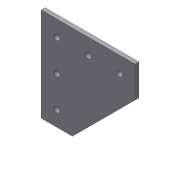
# Autodesk Inventor part: Frame_VerticalAngle_Plate
Saved by Autodesk Inventor 2012 (Build 160160000, 160)
## iProperties
Created: 2012-01-14
Part Number: Frame_VerticalAngle_Plate
Material: Aluminum-6061
Document SubType Name: Modeling
Designer: JesseK
Mass: 38.0914 g
Surface Area: 99.6488 cm^2
Volume: 14.0559 cm^3
Density: 2.71 g/cm^3
Author: JesseK
Autodesk Inventor part; units mm, degrees
ref_plane "YZ Plane" through (0, 0, 0) normal (1, 0, 0) x (0, 1, 0)
ref_plane "XZ Plane" through (0, 0, 0) normal (0, 1, 0) x (-1, 0, 0)
ref_plane "XY Plane" through (0, 0, 0) normal (0, 0, 1) x (1, 0, 0)
sketch "Sketch1" plane through (0, 0, 0) normal (0, 0, 1) x (1, 0, 0)
  line L0 (0, 0) -> (25.4, 0)
  line L1 (25.4, 0) -> (76.2, 50.8)
  line L2 (76.2, 50.8) -> (76.2, 76.2)
  line L3 (76.2, 76.2) -> (0, 76.2)
  line L4 (0, 76.2) -> (0, 0)
  dimension "d0" = 76.2
  dimension "d1" = 76.2
  dimension "d2" = 25.4
  dimension "d3" = 25.4
  constraints: 10 end point, 2 horizontal, 2 vertical
  measures "d0" distance of L2.end L3.end
  measures "d1" distance of L3.end L0.start
  measures "d2" distance of L0.start L0.end
  measures "d3" distance of L1.end L2.end
extrude "Extrusion1" add sketch "Sketch1" along normal blind 3.175
sketch "Sketch2" plane through (0, 0, 3.175) normal (0, 0, 1) x (1, 0, 0)
  line L0 (0, 0) -> (0, 76.2) projected
  line L1 (0, 76.2) -> (76.2, 76.2) projected
  circle A0 centre (12.7, 63.5) radius 2.3813
  dimension "d6" = 4.7625
  dimension "d7" = 12.7
  dimension "d8" = 12.7
  constraints: 1 centre point
  measures "d6" diameter of A0
  measures "d7" distance from line of L1 A0.centre
  measures "d8" distance from line of L0 A0.centre
extrude "Extrusion2" cut sketch "Sketch2" against normal up to next
pattern_linear "Rectangular Pattern1" count 4 spacing 25.4 along (1, 0, 0) of "Extrusion2"
pattern_linear "Rectangular Pattern2" count 4 spacing 25.4 along (0, -1, 0) of "Extrusion2"
body "Solid1"
